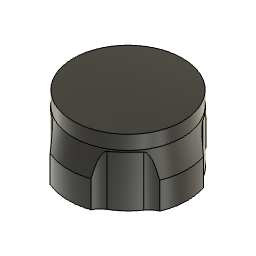
Base-v10 (Autodesk Fusion 360 design; units mm, degrees)
Autodesk Fusion 360 part; units mm, degrees
note: some values were not read from the file. Set by a fixed rule: which sketch regions a step uses.
sketch "Sketch4" plane through (0, 0, 0) normal (0, 0, 1) x (-1, 0, 0)
  circle A0 centre (0, 0) radius 15.7
  arc A1 (6.1849, 14.4304) -> (7.9716, 12.1501) centre (10.6805, 16.1127) ccw
  arc A2 (6.1849, 14.4304) -> (-5.1632, 14.8267) centre (0, 0) ccw
  arc A3 (-7.1047, 12.6765) -> (-5.1632, 14.8267) centre (-9.5305, 16.8184) ccw
  arc A4 (-7.1047, 12.6765) -> (-12.1501, 7.9716) centre (0.8594, -0.9216) ccw
  arc A5 (-14.4304, 6.1849) -> (-12.1501, 7.9716) centre (-16.1127, 10.6805) ccw
  arc A6 (-14.4304, 6.1849) -> (-14.8267, -5.1632) centre (0, 0) ccw
  arc A7 (-12.6765, -7.1047) -> (-14.8267, -5.1632) centre (-16.8184, -9.5305) ccw
  arc A8 (-12.6765, -7.1047) -> (-7.9716, -12.1501) centre (0.9216, 0.8594) ccw
  arc A9 (-6.1849, -14.4304) -> (-7.9716, -12.1501) centre (-10.6805, -16.1127) ccw
  arc A10 (-6.1849, -14.4304) -> (5.1632, -14.8267) centre (0, 0) ccw
  arc A11 (7.1047, -12.6765) -> (5.1632, -14.8267) centre (9.5305, -16.8184) ccw
  arc A12 (7.1047, -12.6765) -> (12.1501, -7.9716) centre (-0.8594, 0.9216) ccw
  arc A13 (14.4304, -6.1849) -> (12.1501, -7.9716) centre (16.1127, -10.6805) ccw
  arc A14 (14.4304, -6.1849) -> (14.8267, 5.1632) centre (0, 0) ccw
  arc A15 (12.6765, 7.1047) -> (14.8267, 5.1632) centre (16.8184, 9.5305) ccw
  arc A16 (12.6765, 7.1047) -> (7.9716, 12.1501) centre (-0.9216, -0.8594) ccw
  dimension "d11" = 31.4
  measures "d11" diameter of A0
sketch "Sketch1" plane through (0, 0, 0) normal (0, 1, 0) x (1, 0, 0)
  line L0 (0, 0) -> (0, -17.25)
  line L1 (0, 0) -> (15.5, 0)
  line L2 (15.5, 0) -> (15.5, -7)
  line L3 (15.5, -7) -> (14.23, -13.605)
  line L4 (14.23, -13.605) -> (14.23, -17.25)
  line L5 (14.23, -17.25) -> (0, -17.25)
  dimension "d1" = 15.5
  dimension "d2" = 14.23
  dimension "d3" = 3.645
  dimension "d4" = 7
  dimension "d5" = 17.25
  constraint coincident L0.start L1.start
  constraint vertical L0
  constraint horizontal L1
  constraint perpendicular L1 L2
  constraint perpendicular L1 L4
  constraint horizontal L5
  measures "d1" distance of L0.start L1.end
  measures "d2" distance of L0.end L4.end
  measures "d3" distance of L3.end L4.end
  measures "d4" distance of L1.end L2.end
  measures "d5" distance of L0.start L0.end
revolve "Revolve1" add sketch "Sketch1" angle 360 about axis through (0, 0, 1.75) along (0, 0, 1)
sketch "Sketch2" plane through (0, 0, 0) normal (0, 0, -1) x (1, 0, 0)
  circle A0 centre (0, 0) radius 15.5
  circle A1 centre (0, 0) radius 9.085
  circle A2 centre (0, 0) radius 12.5
  line L0 (0, 0) -> (26.4938, 0) construction
  line L1 (0, 0) -> (0, 20.2896) construction
  circle A3 centre (9.5305, 16.8184) radius 5
  circle A4 centre (16.1127, 10.6805) radius 5
  line L2 (0, 0) -> (18.26, 19.5815) construction
  line L3 (9.5305, 16.8184) -> (16.1127, 10.6805)
  arc A5 (11.9849, 7.8588) -> (7.0036, 12.504) centre (-0.8594, -0.9216) ccw
  line L4 (12.9405, 20.4752) -> (19.5227, 14.3372)
  dimension "d7" = 18.17
  dimension "d8" = 25
  dimension "d12" = 10
  dimension "d13" = 9
  dimension "d14" = 18.8
  dimension "d24" = 47
  constraint coincident A0.centre A1.centre
  constraint concentric A1 A2
  constraint horizontal L0
  constraint perpendicular L0 L1
  constraint coincident A3.centre L3.start
  constraint coincident A4.centre L3.end
  constraint perpendicular L2 L3
  constraint symmetric A3.centre A4.centre L2
  constraint equal A3 A4
  constraint tangent A4 A5
  constraint coincident A4 A5.start
  constraint coincident A3 A5.end
  constraint coincident A3 L4.start
  constraint coincident A4 L4.end
  constraint perpendicular L2 L4
  constraint tangent A4 L4
  constraint tangent A3 A5
  measures "d7" diameter of A1
  measures "d8" diameter of A2
  measures "d12" diameter of A3
  measures "d13" distance of A3.centre A4.centre
  measures "d14" distance of A0.centre L3
  measures "d24" angle of L0 L2
extrude "Extrude1" cut sketch "Sketch2" against normal blind 2.85 contours A2
extrude "Extrude2" cut sketch "Sketch2" against normal blind 22 contours A0 A4 | A0 A3 A4 | A0 A3 A4 | A0 A3 | A0 A3 A4 A5 | A0 A3 A4 | A3 A4 L4 | A3 A4 L3 | A3 A4 L3 picked at (10.0669, 10.6715)
pattern_circular "C-Pattern1" count 4 over 360 about axis through (0, 0, 1.75) along (0, 0, 1) of "Extrude2"
sketch "Sketch3" plane through (0, 0, 17.25) normal (0, 0, 1) x (-1, 0, 0)
  circle A0 centre (0, 0) radius 13.175
  circle A1 centre (0, 0) radius 14.23
  dimension "d19" = 26.35
  constraint concentric A0 A1
  measures "d19" diameter of A0
extrude "Extrude4" [suppressed]
equation "d1 = ( 31 / 2 ) * 1 mm"
equation "d2 = ( 28.46 / 2 ) * 1 mm"
